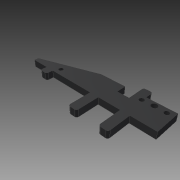
# Autodesk Inventor part: x_motor_upper_nut_stop
Saved by Autodesk Inventor 2014 (Build 180170000, 170)
## iProperties
Created: 2013-12-01
Part Number: x_motor_upper_nut_stop
Material: Plywood, Finish
Document SubType Name: Modeling
Designer: buben
Density: 0.552 g/cm^3
Appearance: Plywood - New
Author: buben
Subject: Laser Cutted
Autodesk Inventor part; units mm, degrees
ref_plane "YZ Plane" through (0, 0, 0) normal (1, 0, 0) x (0, 1, 0)
ref_plane "XZ Plane" through (0, 0, 0) normal (0, 1, 0) x (-1, 0, 0)
ref_plane "XY Plane" through (0, 0, 0) normal (0, 0, 1) x (1, 0, 0)
sketch "Sketch1" plane through (0, 0, 0) normal (0, 0, 1) x (1, 0, 0)
  line L0 (0, 4) -> (0, 0)
  line L1 (0, 0) -> (125, 0)
  line L2 (125, 0) -> (125, 23.5)
  line L3 (57, 23.5) -> (0, 4)
  line L4 (81, 23.5) -> (81, 14.5)
  line L5 (81, 14.5) -> (92, 14.5)
  line L6 (92, 14.5) -> (92, 23.5)
  line L7 (125, 23.5) -> (92, 23.5)
  line L8 (81, 23.5) -> (57, 23.5)
  circle A0 centre (99.5, 19) radius 2.25
  circle A1 centre (119.5, 19) radius 2.25
  circle A2 centre (28.2, 6) radius 2.25
  circle A3 centre (28.2, 6) radius 4.5 construction
  point P0 (92, 19)
  dimension "d0" = 4
  dimension "d1" = 125
  dimension "d2" = 9
  dimension "d3" = 11
  dimension "d4" = 33
  dimension "d5" = 24
  dimension "d6" = 23.5
  dimension "d7" = 4.5
  dimension "d8" = 4.5
  dimension "d9" = 5.5
  dimension "d10" = 20
  dimension "d11" = 4.5
  dimension "d12" = 9
  dimension "d13" = 6
  dimension "d14" = 28.2
  constraints: 18 end point, 6 perpendicular, 4 centre point, 3 parallel, 2 horizontal alignment, 1 coincident, 1 collinear, 1 midpoint, 1 vertical
  measures "d0" distance of L0.start L0.end
  measures "d1" distance of L0.end L1.end
  measures "d2" distance of L5.end L6.end
  measures "d3" distance of L4.end L5.end
  measures "d4" distance of L2.end L6.end
  measures "d5" distance of L4.start L3.start
  measures "d6" distance of L1.end L2.end
  measures "d7" diameter of A1
  measures "d8" diameter of A0
  measures "d9" distance from line of L2 A1.centre
  measures "d10" distance of A1.centre A0.centre
  measures "d11" diameter of A2
  measures "d12" diameter of A3
  measures "d13" distance from line of L1 A2.centre
  measures "d14" distance from line of L0 A2.centre
extrude "Extrusion1" add sketch "Sketch1" along normal blind 6.5
sketch "Sketch2" plane through (0, 0, 6.5) normal (0, 0, 1) x (1, 0, 0)
  line L0 (0, 0) -> (125, 0) projected
  line L1 (125, 23.5) -> (92, 23.5) projected
  line L2 (17, 0) -> (25, 0)
  line L3 (25, 0) -> (25, -4.5)
  line L4 (23, -6.5) -> (19, -6.5)
  line L5 (17, -4.5) -> (17, 0)
  line L6 (96, 0) -> (104, 0)
  line L7 (104, 0) -> (104, -19)
  line L8 (102, -21) -> (98, -21)
  line L9 (96, -19) -> (96, 0)
  line L10 (68, 0) -> (76, 0)
  line L11 (76, 0) -> (76, -19)
  line L12 (74, -21) -> (70, -21)
  line L13 (68, -19) -> (68, 0)
  line L14 (92, 23.5) -> (100, 23.5)
  line L15 (100, 23.5) -> (100, 29.5)
  line L16 (98, 31.5) -> (94, 31.5)
  line L17 (92, 29.5) -> (92, 23.5)
  arc A0 (17, -4.5) -> (19, -6.5) centre (19, -4.5) ccw
  arc A1 (23, -6.5) -> (25, -4.5) centre (23, -4.5) ccw
  arc A2 (96, -19) -> (98, -21) centre (98, -19) ccw
  arc A3 (102, -21) -> (104, -19) centre (102, -19) ccw
  arc A4 (68, -19) -> (70, -21) centre (70, -19) ccw
  arc A5 (74, -21) -> (76, -19) centre (74, -19) ccw
  arc A6 (94, 31.5) -> (92, 29.5) centre (94, 29.5) ccw
  arc A7 (100, 29.5) -> (98, 31.5) centre (98, 29.5) ccw
  line L18 (92, 23.5) -> (92, 14.5) projected
  dimension "d17" = 2
  dimension "d18" = 17
  dimension "d20" = 8
  dimension "d21" = 8
  dimension "d22" = 8
  dimension "d24" = 6.5
  dimension "d25" = 43
  dimension "d26" = 20
  dimension "d29" = 8
  dimension "d40" = 8
  dimension "d41" = 2
  dimension "d42" = 2
  dimension "d45" = 21
  constraints: 32 end point, 16 point on circle, 16 tangent, 8 centre point, 8 parallel, 5 equal radius, 4 horizontal, 4 perpendicular, 4 point on line, 2 collinear
  measures "d17" radius of A0
  measures "d18" distance from line of L5 L0.start
  measures "d20" distance between parallel lines of L3 L5
  measures "d21" distance between parallel lines of L11 L13
  measures "d22" distance between parallel lines of L7 L9
  measures "d24" distance between parallel lines of L0 L4
  measures "d25" distance between parallel lines of L13 L3
  measures "d26" distance between parallel lines of L9 L11
  measures "d29" distance between parallel lines of L15 L17
  measures "d40" distance between parallel lines of L14 L16
  measures "d41" radius of A7
  measures "d42" radius of A6
  measures "d45" distance between parallel lines of L0 L12
sketch "Sketch3" plane through (0, 0, 6.5) normal (0, 0, 1) x (1, 0, 0)
  circle A0 centre (119.5, 19) radius 2.25 projected
  circle A1 centre (109.5, 19.599) radius 2.75
  circle A2 centre (86.5, 19.599) radius 7.5 construction
  dimension "d35" = 5.5
  dimension "d36" = 15
  dimension "d37" = 10
  constraints: 2 centre point, 1 horizontal alignment
  measures "d35" diameter of A1
  measures "d36" diameter of A2
  measures "d37" horizontal distance of A0.centre A1.centre
extrude "Extrusion3" cut sketch "Sketch3" against normal blind 6.5 contours A1
extrude "Extrusion4" add sketch "Sketch2" against normal blind 6.5
body "Solid1"
